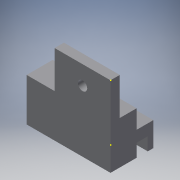
# Autodesk Inventor part: suporte p trilho2
Saved by Autodesk Inventor 2018 (Build 220112000, 112)
## iProperties
Created: 2018-05-30
Part Number: suporte p trilho2
Material: Genérico
Document SubType Name: Modeling
Designer: Ernandes
Density: 1 g/cm^3
Appearance: Padrão
Author: Ernandes
Autodesk Inventor part; units mm, degrees
ref_plane "YZ Plane" through (0, 0, 0) normal (1, 0, 0) x (0, 1, 0)
ref_plane "XZ Plane" through (0, 0, 0) normal (0, 1, 0) x (-1, 0, 0)
ref_plane "XY Plane" through (0, 0, 0) normal (0, 0, 1) x (1, 0, 0)
sketch "Esboço1" plane through (0, 0, 0) normal (1, 0, 0) x (0, 1, 0)
  point P0 (0, 0)
sketch "Esboço2" plane through (0, 0, 0) normal (0, 1, 0) x (-1, 0, 0)
  line L0 (0, 0) -> (0, -20)
  line L1 (0, -20) -> (30, -20)
  line L2 (30, -20) -> (30, 0)
  line L3 (30, 0) -> (0, 0)
  line L4 (15, 0) -> (15, -10)
  circle A0 centre (15, -10) radius 2.5
  dimension "d0" = 20
  dimension "d1" = 30
  dimension "d2" = 5
  constraints: 10 end point, 3 perpendicular, 2 vertical, 1 centre point, 1 coincident, 1 midpoint
  measures "d0" distance of L0.start L0.end
  measures "d1" distance of L0.end L1.end
  measures "d2" diameter of A0
extrude "Extrusão1" add sketch "Esboço2" along normal blind 5
sketch "Esboço3" plane through (0, 0, 0) normal (0, -1, 0) x (1, 0, 0)
  line L0 (0, 0) -> (0, -20) projected
  line L1 (0, -20) -> (0, -43)
  line L2 (0, -43) -> (-45, -43)
  line L3 (-45, -43) -> (-45, -20)
  line L4 (0, -20) -> (-30, -20) projected
  line L5 (-45, -20) -> (0, -20)
  dimension "d5" = 23
  dimension "d6" = 45
  constraints: 8 end point, 3 perpendicular, 1 vertical
  measures "d5" distance of L0.end L1.end
  measures "d6" distance of L1.end L2.end
extrude "Extrusão2" add sketch "Esboço3" against normal blind 14
sketch "Esboço4" plane through (0, 14, 0) normal (0, 1, 0) x (1, 0, 0)
  line L0 (0, 0) -> (0, 43) projected
  line L1 (0, 43) -> (0, 36)
  line L2 (0, 36) -> (0, 30)
  line L3 (0, 30) -> (-45, 30)
  line L4 (-45, 43) -> (-45, 20) projected
  line L5 (-45, 30) -> (-45, 36)
  line L6 (-45, 36) -> (0, 36)
  dimension "d9" = 7
  dimension "d10" = 6
  constraints: 10 end point, 3 point on line, 2 perpendicular, 1 vertical
  measures "d9" distance of L0.end L1.end
  measures "d10" distance of L1.end L2.end
extrude "Extrusão3" add sketch "Esboço4" along normal blind 9
sketch "Esboço5" plane through (-45, 14, -30) normal (0, 0, 1) x (1, 0, 0)
  point P0 (45, -14)
sketch "Esboço6" plane through (0, 14, -36) normal (0, 0, -1) x (-1, 0, 0)
  line L0 (45, 9) -> (0, 9) projected
  line L1 (0, 9) -> (45, 9)
  line L2 (45, 9) -> (45, 6)
  line L3 (45, 0) -> (45, 9) projected
  line L4 (45, 6) -> (0, 6)
  line L5 (0, 0) -> (0, 9) projected
  line L6 (0, 6) -> (0, 9)
  point P0 (0, -14)
  dimension "d13" = 3
  constraints: 8 end point, 2 collinear, 1 parallel, 1 point on line
  measures "d13" distance of L0.start L2.end
extrude "Extrusão4" add sketch "Esboço6" along normal blind 7
sketch "Esboço7" plane through (-45, 0, -43) normal (-1, 0, 0) x (0, 0, 1)
  line L0 (23, 14) -> (13, 14) projected
  line L1 (13, 14) -> (10.3, 14)
  line L2 (10.3, 14) -> (10.3, 9.5)
  line L3 (10.3, 9.5) -> (13, 9.5)
  line L4 (13, 9.5) -> (13, 14)
  point P0 (43, 0)
  dimension "d16" = 2.7
  dimension "d17" = 4.5
  constraints: 8 end point, 3 perpendicular, 1 horizontal
  measures "d16" distance of L0.end L1.end
  measures "d17" distance of L1.end L2.end
extrude "Extrusão5" add sketch "Esboço7" along normal blind 10
move faces "Mover1" translate (10, 0, 0) faces at (-55, 12.5, -31.8)
sketch "Esboço8" plane through (0, 5, 0) normal (0, 1, 0) x (1, 0, 0)
  line L0 (-30, 0) -> (0, 0) projected
  line L1 (-15, 0) -> (-15, 10)
  circle A0 centre (-15, 10) radius 2.5
  dimension "d23" = 10
  constraints: 2 end point, 1 centre point, 1 coincident, 1 midpoint, 1 vertical
  measures "d23" distance of L1.start L1.end
extrude "Extrusão6" add sketch "Esboço8" against normal blind 5
sketch "Esboço9" plane through (0, 5, 0) normal (0, 1, 0) x (1, 0, 0)
  line L0 (-30, 0) -> (0, 0) projected
  line L1 (0, 0) -> (-10, 0)
  line L2 (-10, 0) -> (-20, 0)
  line L3 (-20, 0) -> (-20, 10)
  line L4 (-10, 0) -> (-10, 10)
  circle A0 centre (-10, 10) radius 2.5
  circle A1 centre (-20, 10) radius 2.5
  dimension "d26" = 10
  dimension "d27" = 10
  dimension "d28" = 10
  dimension "d29" = 10
  dimension "d30" = 5
  dimension "d31" = 5
  constraints: 8 end point, 2 centre point, 2 coincident, 2 perpendicular, 2 point on line
  measures "d26" distance of L0.end L1.end
  measures "d27" distance of L1.end L2.end
  measures "d28" distance of L2.end L3.end
  measures "d29" distance of L1.end L4.end
  measures "d30" diameter of A0
  measures "d31" diameter of A1
extrude "Extrusão7" cut sketch "Esboço9" against normal blind 5
